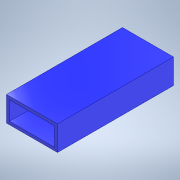
# Autodesk Inventor part: Electronics Lid
Saved by Autodesk Inventor 2022 (Build 260153000, 153)
## iProperties
Created: 2022-08-13
Part Number: Electronics Lid
Material: Generic
Document SubType Name: Modeling
Designer: Nick
Density: 1 g/cm^3
Appearance: Blue - Wall Paint - Glossy
Author: Nick
Autodesk Inventor part; units mm, degrees
ref_plane "YZ Plane" through (0, 0, 0) normal (1, 0, 0) x (0, 1, 0)
ref_plane "XZ Plane" through (0, 0, 0) normal (0, 1, 0) x (-1, 0, 0)
ref_plane "XY Plane" through (0, 0, 0) normal (0, 0, 1) x (1, 0, 0)
sketch "Sketch1" plane through (0, 0, 0) normal (0, 0, 1) x (1, 0, 0)
  line L0 (0, 0) -> (33, 0)
  line L1 (33, 0) -> (33, 2)
  line L2 (33, 2) -> (0, 2)
  line L3 (0, 2) -> (0, 0)
  line L4 (0, 16) -> (33, 16)
  line L5 (33, 16) -> (33, 14)
  line L6 (33, 14) -> (0, 14)
  line L7 (0, 14) -> (0, 16)
  line L8 (33, 14) -> (31, 14)
  line L9 (31, 14) -> (31, 2)
  line L10 (31, 2) -> (33, 2)
  line L11 (33, 2) -> (33, 14)
  line L12 (0, 14) -> (2, 14)
  line L13 (2, 14) -> (2, 2)
  line L14 (2, 2) -> (0, 2)
  line L15 (0, 2) -> (0, 14)
  point P0 (31, 2)
  point P1 (2, 2)
  dimension "d0" = 2
  dimension "d1" = 12
  dimension "d2" = 29
  dimension "d5" = 2
  dimension "d6" = 2
  constraints: 32 end point, 8 parallel, 4 horizontal, 4 perpendicular, 1 collinear
  measures "d0" distance of L0.end L1.end
  measures "d1" distance of L8.end L9.end
  measures "d2" distance between parallel lines of L9 L13
  measures "d5" distance between parallel lines of L11 L9
  measures "d6" distance between parallel lines of L15 L13
extrude "Extrusion1" add sketch "Sketch1" along normal blind 75 contours L3 L2 L1 L0 | L15 L6 L13 L2 | L2 L9 L6 L11 | L7 L4 L5 L6
body "Solid1"
